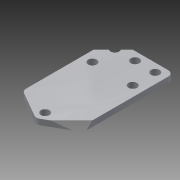
# Autodesk Inventor part: Roller Pneumatic Back Connector (Custom)
Saved by Autodesk Inventor 2014 (Build 180170000, 170)
## iProperties
Created: 2014-01-06
Part Number: Roller Pneumatic Back Connector (Custom)
Material: Aluminum 6061
Document SubType Name: Modeling
Designer: Andrew Toennies
Density: 7.85 g/cm^3
Appearance: Aluminum - Flat
Mass: 11.2814 g
Surface Area: 21.4027 cm^2
Volume: 1.43712 cm^3
Author: Andrew Toennies
Autodesk Inventor part; units mm, degrees
ref_plane "YZ Plane" through (0, 0, 0) normal (1, 0, 0) x (0, 1, 0)
ref_plane "XZ Plane" through (0, 0, 0) normal (0, 1, 0) x (-1, 0, 0)
ref_plane "XY Plane" through (0, 0, 0) normal (0, 0, 1) x (1, 0, 0)
sketch "Sketch1" plane through (0, 0, 0) normal (0, 1, 0) x (-1, 0, 0)
  circle A0 centre (0, 0) radius 2.413
  circle A1 centre (0, 50.8) radius 2.413
  line L0 (0, 50.8) -> (0, 0) construction
  circle A2 centre (11.3919, 12.7) radius 2.413
  circle A3 centre (11.3919, 0) radius 2.413
  circle A4 centre (-11.3919, 0) radius 2.413
  circle A5 centre (-11.3919, 12.7) radius 2.413
  line L1 (-11.3919, 0) -> (-11.3919, 12.7) construction
  line L2 (-11.3919, 12.7) -> (11.3919, 12.7) construction
  line L3 (1.5875, 55.2652) -> (15.5575, 47.1996)
  line L4 (-15.5575, 47.1996) -> (-1.5875, 55.2652)
  arc A6 (1.5875, 55.2652) -> (-1.5875, 55.2652) centre (0, 52.5156) ccw
  arc A7 (-15.5575, 47.1996) -> (-17.145, 44.45) centre (-13.97, 44.45) ccw
  arc A8 (17.145, 44.45) -> (15.5575, 47.1996) centre (13.97, 44.45) ccw
  line L5 (-17.145, 6.35) -> (-17.145, 44.45)
  line L6 (17.145, -4.7625) -> (17.145, 44.45)
  line L7 (17.145, -4.7625) -> (-17.145, -4.7625)
  line L8 (-17.145, 6.35) -> (-17.145, -4.7625)
  line L9 (13.97, 44.45) -> (-13.97, 44.45) construction
  point P0 (0, 25.4)
  point P1 (0, 56.1818)
  point P2 (26.6578, 40.7909)
  point P3 (26.6578, 10.0091)
  point P4 (-26.6578, 10.0091)
  point P5 (-26.6578, 40.7909)
  dimension "d1" = 4.826
  dimension "d2" = 50.8
  dimension "d3" = 4.826
  dimension "d4" = 4.826
  dimension "d5" = 12.7
  dimension "d6" = 11.3919
  dimension "d7" = 11.3919
  dimension "d8" = 0
  dimension "d9" = 4.826
  dimension "d10" = 4.826
  dimension "d11" = 11.3919
  dimension "d12" = 12.7
  dimension "d14" = 3.175
  dimension "d17" = 38.1
  dimension "d18" = 34.29
  dimension "d19" = 4.7625
  dimension "d20" = 6.35
  dimension "d21" = 49.2125
  dimension "d22" = 8.0656
  constraints: 20 end point, 9 centre point, 6 point on circle, 6 tangent, 5 point on line, 4 perpendicular, 2 equal radius, 2 parallel, 1 coincident, 1 midpoint, 1 vertical, 7 other
  measures "d1" diameter of A1
  measures "d2" distance of L0.start L0.end
  measures "d3" diameter of A2
  measures "d4" diameter of A3
  measures "d5" distance of A3.centre L2.end
  measures "d6" distance from line of L0 A3.centre
  measures "d7" distance from line of L0 L2.end
  measures "d8" vertical distance of point (0, 0) A3.centre
  measures "d9" diameter of A4
  measures "d10" diameter of A5
  measures "d11" distance between parallel lines of L1 L0
  measures "d12" distance of L1.start L1.end
  measures "d14" radius of A6
  measures "d17" distance of L5.start L5.end
  measures "d18" distance between parallel lines of L6 L5
  measures "d19" distance from line of point (0, 0) L7
  measures "d20" vertical distance of L5.start L0.end
  measures "d21" distance of L6.start L6.end
  measures "d22" vertical distance of L5.end A6.centre
extrude "Extrusion1" add sketch "Sketch1" along normal blind 3.175
fillet "Fillet1" radius 3.175 2 edges at (-17.145, 1.5875, -4.7625) (17.145, 1.5875, -4.7625)
equation "\"d7\" = d6"
equation "\"d11\" = d6"
equation "\"d21\" = d20 + d19 + d17"
body "Solid1"
